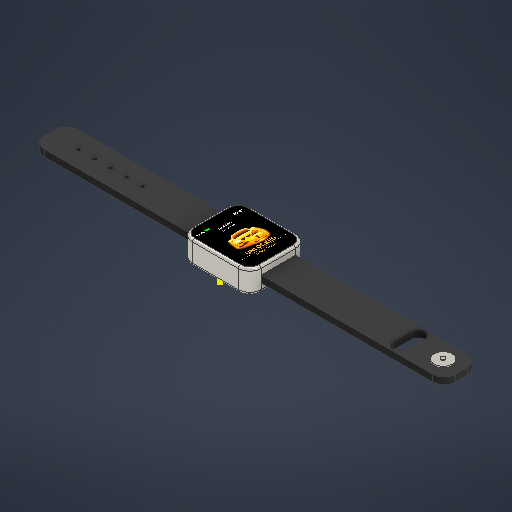
# Autodesk Inventor part: Design Display Unlock
Saved by Autodesk Inventor 2027 (Build 310192000, 192)
## iProperties
Created: 2026-05-31
Part Number: Design Display Unlock
Material: Generic
Document SubType Name: Sheet Metal
Designer: acer
Density: 1 g/cm^3
Sheet Metal Rule: Default_mm
Appearance: Default
Author: acer
Autodesk Inventor part; units mm, degrees
ref_plane "YZ Plane" through (0, 0, 0) normal (1, 0, 0) x (0, 1, 0)
ref_plane "XZ Plane" through (0, 0, 0) normal (0, 1, 0) x (-1, 0, 0)
ref_plane "XY Plane" through (0, 0, 0) normal (0, 0, 1) x (1, 0, 0)
sketch "Sketch1" plane through (0, 0, 0) normal (0, 1, 0) x (-1, 0, 0)
  line L0 (17.2059, 11.8382) -> (-12.7941, 11.8382)
  line L1 (-12.7941, 11.8382) -> (-12.7941, -13.1618)
  line L2 (-12.7941, -13.1618) -> (17.2059, -13.1618)
  line L3 (17.2059, -13.1618) -> (17.2059, 11.8382)
  point P0 (0, 0)
  dimension "d0" = 25
  dimension "d1" = 30
  constraints: 8 end point, 2 parallel, 1 horizontal, 1 perpendicular
  measures "d0" distance of L2.end L0.start
  measures "d1" distance between parallel lines of L3 L1
extrude "Extrusion1" add sketch "Sketch1" along normal blind 10
fillet "Fillet1" radius 5 1 edges at (12.7941, 5, 11.8382)
sketch "Sketch2" plane through (12.7941, 0, -13.1618) normal (0, 0, -1) x (-1, 0, 0)
  point P0 (12.7941, 0)
fillet "Fillet2" radius 5 1 edges at (12.7941, 5, -13.1618)
fillet "Fillet3" radius 5 1 edges at (-17.2059, 5, -13.1618)
fillet "Fillet4" radius 5 1 edges at (-17.2059, 5, 11.8382)
fillet "Fillet5" radius 1 8 edges at (-15.7414, 10, -11.6973) (-2.2059, 10, -13.1618) (11.3297, 10, -11.6973) (12.7941, 10, -0.6618) (11.3297, 10, 10.3738) (-2.2059, 10, 11.8382) (-15.7414, 10, 10.3738) (-17.2059, 10, -0.6618)
fillet "Fillet6" radius 1 8 edges at (-17.2059, 0, -0.6618) (-15.7414, 0, 10.3738) (-2.2059, 0, 11.8382) (11.3297, 0, 10.3738) (12.7941, 0, -0.6618) (11.3297, 0, -11.6973) (-2.2059, 0, -13.1618) (-15.7414, 0, -11.6973)
sketch "Sketch3" plane through (12.7941, 9, 6.8382) normal (1, 0, 0) x (0, 0, -1)
  line L0 (15, 0) -> (15, -8) projected
  line L1 (0, -8) -> (0, 0) projected
  line L2 (15, -5.5) -> (0, -5.5)
  line L3 (0, -5.5) -> (0, -2.5)
  line L4 (0, -2.5) -> (15, -2.5)
  line L5 (15, -2.5) -> (15, -5.5)
  line L6 (0, 0) -> (15, 0) projected
  point P0 (6.8382, -9)
  point P1 (7.5, -2.5)
  point P2 (7.5, 0)
  point P3 (15, -2.5)
  point P4 (0, -5.5)
  dimension "d10" = 3
  dimension "d11" = 2.5
  constraints: 8 end point, 2 midpoint, 2 parallel, 2 point on line, 1 horizontal, 1 perpendicular
  measures "d10" distance between parallel lines of L2 L4
  measures "d11" distance of point (7.5, -2.5) point (7.5, 0)
extrude "Extrusion2" add sketch "Sketch3" along normal blind 80 contours L0 L2 L1 L4
sketch "Sketch4" plane through (-17.2059, 9, -8.1618) normal (-1, 0, 0) x (0, 0, 1)
  line L0 (14.6937, -5.5) -> (0, -5.5)
  line L1 (0, -5.5) -> (0, -2.5)
  line L2 (0, -2.5) -> (14.6937, -2.5)
  line L3 (14.6937, -2.5) -> (14.6937, -5.5)
  line L4 (0, 0) -> (15, 0) projected
  point P0 (8.1618, -9)
  dimension "d14" = 2.5
  dimension "d15" = 3
  constraints: 8 end point, 2 parallel, 1 horizontal, 1 perpendicular
  measures "d14" distance between parallel lines of L2 L4
  measures "d15" distance between parallel lines of L0 L2
extrude "Extrusion3" add sketch "Sketch4" along normal blind 70
fillet "Fillet7" radius 5 1 edges at (-87.2059, 5, -8.1618)
fillet "Fillet8" radius 5 1 edges at (-87.2059, 5, 6.5319)
fillet "Fillet9" radius 5 1 edges at (92.7941, 5, 6.8382)
fillet "Fillet10" radius 5 1 edges at (92.7941, 5, -8.1618)
sketch "Sketch5" plane through (7.7941, 9, -13.1618) normal (0, 0, -1) x (-1, 0, 0)
  line L0 (18, -4) -> (12, -4) construction
  line L1 (18, -6) -> (12, -6)
  line L2 (12, -2) -> (18, -2)
  arc A0 (18, -6) -> (18, -2) centre (18, -4) ccw
  arc A1 (12, -2) -> (12, -6) centre (12, -4) ccw
  line L3 (20, -8) -> (0, -8) projected
  line L4 (0, 0) -> (20, 0) projected
  line L5 (20, 0) -> (20, -8) projected
  line L6 (0, -8) -> (0, 0) projected
  point P0 (7.7941, -9)
  point P1 (15, -4)
  point P2 (15, -6)
  point P3 (15, -2)
  point P4 (10, -4)
  point P5 (0, -4)
  dimension "d22" = 2
  dimension "d23" = 2
  dimension "d24" = 2
  dimension "d25" = 10
  constraints: 8 end point, 5 point on circle, 4 midpoint, 4 tangent, 2 centre point, 1 horizontal, 1 parallel
  measures "d22" distance from line of L3 point (15, -6)
  measures "d23" distance from line of point (15, -2) L4
  measures "d24" distance from line of L5 L0.start
  measures "d25" distance of point (10, -4) point (0, -4)
extrude "Extrusion4" add sketch "Sketch5" along normal blind 0.5 contours L1 A1 L2 A0
sketch "Sketch6" plane through (-17.2059, 6.5, 6.5319) normal (0, 1, 0) x (1, 0, 0)
  line L0 (87, 0.1937) -> (87, 14.1937) construction
  line L1 (84, 3.1937) -> (84, 11.1937)
  line L2 (90, 11.1937) -> (90, 3.1937)
  arc A0 (84, 3.1937) -> (90, 3.1937) centre (87, 3.1937) ccw
  arc A1 (90, 11.1937) -> (84, 11.1937) centre (87, 11.1937) ccw
  line L3 (110, 9.6937) -> (110, 4.6937) projected
  line L4 (30, 14.6937) -> (105, 14.6937) projected
  line L5 (30, -0.3063) -> (105, -0.3063) projected
  line L6 (29, 14.6937) -> (29, -0.3063) projected
  point P0 (17.2059, 6.5319)
  point P1 (87, 7.1937)
  point P2 (110, 7.1937)
  point P3 (90, 7.1937)
  point P4 (29, 7.1937)
  point P5 (84, 7.1937)
  dimension "d28" = 20
  dimension "d29" = 0.5
  dimension "d30" = 0.5
  dimension "d31" = 55
  constraints: 8 end point, 7 point on circle, 5 midpoint, 4 tangent, 2 centre point, 2 point on line, 1 parallel, 1 vertical
  measures "d28" distance of point (110, 7.194) point (90, 7.194)
  measures "d29" distance from line of L0.end L4
  measures "d30" distance from line of point (87, 0.194) L5
  measures "d31" distance of point (29, 7.194) point (84, 7.194)
extrude "Extrusion5" cut sketch "Sketch6" against normal blind 10000
sketch "Sketch7" plane through (12.7941, 6.5, 6.8382) normal (0, 1, 0) x (1, 0, 0)
  circle A0 centre (72, 7.5) radius 3.9925
  line L0 (80, 10) -> (80, 5) projected
  line L1 (0, 0) -> (75, 0) projected
  point P0 (-12.7941, 6.8382)
  point P1 (80, 7.5)
  dimension "d34" = 8
  dimension "d35" = 7.5
  constraints: 1 centre point, 1 midpoint
  measures "d34" distance of A0.centre point (80, 7.5)
  measures "d35" distance from line of L1 A0.centre
extrude "Extrusion6" add sketch "Sketch7" along normal blind 0.5
sketch "Sketch8" plane through (84.7941, 7, -0.6618) normal (0, 1, 0) x (1, 0, 0)
  circle A0 centre (0, 0) radius 0.939
  point P0 (-84.7941, -0.6618)
  constraints: 1 centre point
extrude "Extrusion7" add sketch "Sketch8" along normal blind 0.5
sketch "Sketch9" plane through (-17.2059, 6.5, 6.5319) normal (0, 1, 0) x (1, 0, 0)
  circle A0 centre (-29.4386, 7.3) radius 0.9829
  line L0 (0, 0) -> (-65, 0) projected
  point P0 (17.2059, 6.5319)
  dimension "d40" = 7.3
  constraints: 1 centre point
  measures "d40" distance from line of L0 A0.centre
extrude "Extrusion8" cut sketch "Sketch9" against normal blind 10
sketch "Sketch10" plane through (-17.2059, 6.5, 6.5319) normal (0, 1, 0) x (1, 0, 0)
  circle A0 centre (-36.4386, 7.3) radius 0.953
  line L0 (0, 0) -> (-65, 0) projected
  circle A1 centre (-29.4386, 7.3) radius 0.9829 projected
  point P0 (17.2059, 6.5319)
  dimension "d43" = 7.3
  dimension "d44" = 7
  constraints: 1 centre point
  measures "d43" distance from line of L0 A0.centre
  measures "d44" distance of A1.centre A0.centre
extrude "Extrusion9" cut sketch "Sketch10" against normal blind 10 contours A0
sketch "Sketch11" plane through (-17.2059, 6.5, 6.5319) normal (0, 1, 0) x (1, 0, 0)
  circle A0 centre (-43.4386, 7.3) radius 0.953
  line L0 (0, 0) -> (-65, 0) projected
  circle A1 centre (-36.4386, 7.3) radius 0.953 projected
  point P0 (17.2059, 6.5319)
  dimension "d47" = 7.3
  dimension "d48" = 7
  constraints: 1 centre point
  measures "d47" distance from line of L0 A0.centre
  measures "d48" distance of A1.centre A0.centre
extrude "Extrusion10" cut sketch "Sketch11" against normal blind 10 contours A0
sketch "Sketch12" plane through (-17.2059, 6.5, 6.5319) normal (0, 1, 0) x (1, 0, 0)
  circle A0 centre (-50.4386, 7.3) radius 0.9406
  line L0 (0, 0) -> (-65, 0) projected
  circle A1 centre (-43.4386, 7.3) radius 0.953 projected
  point P0 (17.2059, 6.5319)
  dimension "d51" = 7.3
  dimension "d52" = 7
  constraints: 1 centre point
  measures "d51" distance from line of L0 A0.centre
  measures "d52" distance of A0.centre A1.centre
extrude "Extrusion11" cut sketch "Sketch12" against normal blind 10 contours A0
sketch "Sketch13" plane through (-17.2059, 6.5, 6.5319) normal (0, 1, 0) x (1, 0, 0)
  circle A0 centre (-57.4386, 7.3) radius 0.983
  line L0 (0, 0) -> (-65, 0) projected
  circle A1 centre (-50.4386, 7.3) radius 0.9406 projected
  point P0 (17.2059, 6.5319)
  dimension "d55" = 7.3
  dimension "d56" = 7
  constraints: 1 centre point
  measures "d55" distance from line of L0 A0.centre
  measures "d56" distance of A0.centre A1.centre
extrude "Extrusion12" cut sketch "Sketch13" against normal blind 10 contours A0
sketch "Sketch14" plane through (12.7941, 1, 6.8382) normal (1, 0, 0) x (0, 0, -1)
  point P0 (6.8382, -1)
sketch "Sketch15" plane through (-12.2059, 9, 11.8382) normal (0, 0, 1) x (1, 0, 0)
  point P0 (12.2059, -9)
sketch "Sketch16" plane through (0, 0, 0) normal (0, -1, 0) x (1, 0, 0)
  point P0 (0, 0)
sketch "Sketch17" plane through (0, 10, 0) normal (0, 1, 0) x (1, 0, 0)
  point P0 (0, 0)
sketch "Sketch18" plane through (0, 0, 0) normal (0, -1, 0) x (1, 0, 0)
  line L0 (-12.9559, -4.6618) -> (-12.9559, 3.3382) construction
  line L1 (-14.2059, -3.4118) -> (-14.2059, 2.0882)
  line L2 (-11.7059, 2.0882) -> (-11.7059, -3.4118)
  arc A0 (-14.2059, -3.4118) -> (-11.7059, -3.4118) centre (-12.9559, -3.4118) ccw
  arc A1 (-11.7059, 2.0882) -> (-14.2059, 2.0882) centre (-12.9559, 2.0882) ccw
  line L3 (-16.2059, -8.1618) -> (-16.2059, 6.8382) projected
  line L4 (7.7941, -12.1618) -> (-12.2059, -12.1618) projected
  line L5 (-12.2059, 10.8382) -> (7.7941, 10.8382) projected
  circle A2 centre (-12.9559, -3.4118) radius 0.75
  circle A3 centre (-12.9559, 2.0882) radius 0.75
  circle A4 centre (-12.9559, -1.4118) radius 0.45
  circle A5 centre (-12.9559, 0.0882) radius 0.45
  point P0 (0, 0)
  point P1 (-12.9559, -0.6618)
  dimension "d59" = 2
  dimension "d60" = 7.5
  dimension "d61" = 7.5
  dimension "d62" = 2.5
  dimension "d63" = 1.5
  dimension "d64" = 1.5
  dimension "d65" = 0.9
  dimension "d66" = 0.9
  dimension "d67" = 0.8
  dimension "d68" = 0.8
  dimension "d69" = 0.6
  constraints: 8 end point, 7 point on circle, 6 centre point, 4 point on line, 4 tangent, 2 coincident, 1 midpoint, 1 parallel, 1 vertical
  measures "d59" distance between parallel lines of L1 L3
  measures "d60" distance from line of L4 point (-12.956, -4.662)
  measures "d61" distance from line of L5 L0.end
  measures "d62" distance between parallel lines of L2 L1
  measures "d63" diameter of A2
  measures "d64" diameter of A3
  measures "d65" diameter of A5
  measures "d66" diameter of A4
extrude "Extrusion13" cut sketch "Sketch18" against normal blind 0.1
sketch "Sketch19" plane through (0, 0, 0) normal (0, -1, 0) x (1, 0, 0)
  circle A0 centre (-1.2059, -0.6618) radius 8.0816
  line L0 (11.7941, 6.8382) -> (11.7941, -8.1618) projected
  line L1 (-12.2059, 10.8382) -> (7.7941, 10.8382) projected
  point P0 (0, 0)
  dimension "d72" = 13
  dimension "d73" = 11.5
  constraints: 1 centre point
  measures "d72" distance from line of L0 A0.centre
  measures "d73" distance from line of L1 A0.centre
extrude "Extrusion14" add sketch "Sketch19" along normal blind 0.3
fillet "Fillet11" radius 1 1 edges at (-9.2875, -0.3, -0.6618)
sketch "Sketch20" plane through (0, 10, 0) normal (0, 1, 0) x (1, 0, 0)
  line L0 (-5.8471, 13.2923) -> (28.3198, 13.2923) construction
  line L1 (28.3198, 13.2923) -> (28.3198, -11.3008) construction
  line L2 (28.3198, -11.3008) -> (-5.8471, -11.3008) construction
  line L3 (-5.8471, -11.3008) -> (-5.8471, 13.2923) construction
  point P0 (0, 0)
  constraints: 2 other
decal "Decal1"
sketch "Sketch21" plane through (0, 10, 0) normal (0, 1, 0) x (1, 0, 0)
  line L0 (-19.6965, 13.304) -> (-5.6469, 13.304) construction
  line L1 (-5.6469, 13.304) -> (-5.6469, -11.696) construction
  line L2 (-5.6469, -11.696) -> (-19.6965, -11.696) construction
  line L3 (-19.6965, -11.696) -> (-19.6965, 13.304) construction
  point P0 (0, 0)
  point P1 (-12.6717, 13.304)
  point P2 (-12.6717, -11.696)
  dimension "d113" = 25
  constraints: 2 midpoint, 2 other
  measures "d113" distance of point (-12.672, 13.304) point (-12.672, -11.696)
decal "Decal2"
sketch "Sketch22" plane through (0, 10, 0) normal (0, 1, 0) x (1, 0, 0)
  line L0 (-13.8359, 12.0798) -> (73.322, 12.0798) construction
  line L1 (73.322, 12.0798) -> (73.322, -10.9202) construction
  line L2 (73.322, -10.9202) -> (-13.8359, -10.9202) construction
  line L3 (-13.8359, -10.9202) -> (-13.8359, 12.0798) construction
  point P0 (0, 0)
  dimension "d122" = 23
  constraints: 2 other
  measures "d122" distance between parallel lines of L0 L2
decal "Decal3"
equation "\"BendRadius\" = Thickness"
equation "\"BendReliefWidth\" = Thickness"
equation "\"BendReliefDepth\" = 0.5 * Thickness"
equation "\"CornerReliefSize\" = 4 * Thickness"
equation "\"MinimumRemnant\" = 2 * Thickness"
equation "\"TransitionRadius\" = BendRadius"
equation "\"JacobiRadiusSize\" = BendRadius"
equation "\"GapSize\" = Thickness"
equation "\"Thickness\" = 0.5"
body "Solid1"
